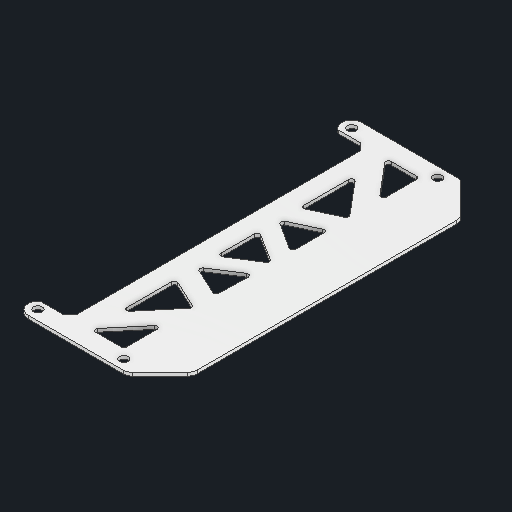
# Autodesk Inventor part: ramp
Saved by Autodesk Inventor 2025 (Build 290162000, 162)
## iProperties
Created: 2024-08-22
Part Number: ramp
Material: Acetal Resin, White
Document SubType Name: Sheet Metal
Designer: averey
Density: 1.425 g/cm^3
Appearance: Smooth - White
Flat Pattern Width: 6.82628 cm
Flat Pattern Length: 16.0338 cm
Flat Pattern Area: 109.451 cm^2
Sheet Metal Rule: Default
Sheet Metal Width: 2.688 in
Sheet Metal Length: 6.313 in
Sheet Metal Area: 16.965 in^2
Author: averey
Autodesk Inventor part; units mm, degrees
ref_plane "YZ Plane" through (0, 0, 0) normal (1, 0, 0) x (0, 1, 0)
ref_plane "XZ Plane" through (0, 0, 0) normal (0, 1, 0) x (-1, 0, 0)
ref_plane "XY Plane" through (0, 0, 0) normal (0, 0, 1) x (1, 0, 0)
sketch "Sketch1" plane through (0, 0, 0) normal (0, 1, 0) x (-1, 0, 0)
  circle A0 centre (0, 0) radius 2.0955
  circle A1 centre (41.2753, 0) radius 2.0955
  circle A2 centre (0, -150.8125) radius 2.0955
  circle A3 centre (41.2753, -150.8125) radius 2.0955
  arc A4 (43.9079, -3.9688) -> (41.2753, 4.7625) centre (41.2753, 0) ccw
  arc A5 (41.2753, -155.575) -> (43.9079, -146.8438) centre (41.2753, -150.8125) ccw
  line L0 (29.8453, -7.366) -> (29.8453, -143.4465)
  line L1 (41.2753, -155.575) -> (0, -155.575)
  line L2 (0, 4.7625) -> (41.2753, 4.7625)
  line L3 (33.2426, -3.9688) -> (29.8453, -7.366)
  line L4 (29.8453, -143.4465) -> (33.2426, -146.8438)
  line L5 (17.9778, -146.431) -> (5.6515, -146.431)
  line L6 (5.6515, -4.3815) -> (17.9778, -4.3815)
  line L7 (18.9507, -6.4678) -> (6.6244, -21.1577)
  line L8 (20.7013, -4.3815) -> (39.8776, -4.3815) construction
  line L9 (18.4584, -21.28) -> (5.4454, -36.7883)
  line L10 (5.8815, -38.7557) -> (18.8946, -44.8238)
  line L11 (4.3815, -38.0562) -> (18.7398, -38.0562) construction
  line L12 (18.6151, -54.7828) -> (6.3567, -49.0665)
  line L13 (6.1698, -65.111) -> (18.7659, -57.0016)
  line L14 (18.9507, -144.3447) -> (6.6244, -129.6548)
  line L15 (20.7013, -146.431) -> (39.8776, -146.431) construction
  line L16 (18.4584, -129.5325) -> (5.4454, -114.0242)
  line L17 (5.8815, -112.0568) -> (18.8946, -105.9887)
  line L18 (4.3815, -112.7563) -> (18.7398, -112.7563) construction
  line L19 (18.6151, -96.0297) -> (6.1882, -101.8245)
  line L20 (18.7659, -93.8109) -> (6.339, -85.8105)
  line L21 (20.7013, -95.0569) -> (35.4808, -95.0569) construction
  line L22 (6.0792, -76.4797) -> (18.7526, -84.4929)
  line L23 (6.0792, -74.3328) -> (18.7526, -66.3196)
  line L24 (4.3815, -20.3414) -> (4.3815, -5.6515)
  line L25 (20.7013, -22.0963) -> (20.7013, -43.6728)
  line L26 (4.2127, -64.0121) -> (4.5503, -50.1866)
  line L27 (20.7013, -67.3931) -> (20.7013, -83.4194)
  line L28 (20.7013, -107.1397) -> (20.7013, -128.7162)
  line L29 (4.3815, -145.161) -> (4.3815, -130.4711)
  line L30 (4.3815, -100.6735) -> (4.3815, -86.8783)
  arc A6 (4.3815, -20.3414) -> (6.6244, -21.1577) centre (5.6515, -20.3414) ccw
  arc A7 (5.6515, -4.3815) -> (4.3815, -5.6515) centre (5.6515, -5.6515) ccw
  arc A8 (18.9507, -6.4678) -> (17.9778, -4.3815) centre (17.9778, -5.6515) ccw
  arc A9 (20.7013, -22.0963) -> (18.4584, -21.28) centre (19.4313, -22.0963) ccw
  arc A10 (5.4454, -36.7883) -> (5.8815, -38.7557) centre (6.4183, -37.6047) ccw
  arc A11 (18.8946, -44.8238) -> (20.7013, -43.6728) centre (19.4313, -43.6728) ccw
  arc A12 (6.3567, -49.0665) -> (4.5503, -50.1866) centre (5.8199, -50.2176) ccw
  arc A13 (4.2127, -64.0121) -> (6.1698, -65.111) centre (5.4823, -64.0431) ccw
  arc A14 (18.7659, -57.0016) -> (18.6151, -54.7828) centre (18.0784, -55.9338) ccw
  arc A15 (6.0792, -74.3328) -> (6.0792, -76.4797) centre (6.7579, -75.4063) ccw
  arc A16 (18.7526, -84.4929) -> (20.7013, -83.4194) centre (19.4313, -83.4194) ccw
  arc A17 (20.7013, -67.3931) -> (18.7526, -66.3196) centre (19.4313, -67.3931) ccw
  arc A18 (6.339, -85.8105) -> (4.3815, -86.8783) centre (5.6515, -86.8783) ccw
  arc A19 (18.6151, -96.0297) -> (18.7659, -93.8109) centre (18.0784, -94.8787) ccw
  arc A20 (4.3815, -100.6735) -> (6.1882, -101.8245) centre (5.6515, -100.6735) ccw
  arc A21 (20.7013, -107.1397) -> (18.8946, -105.9887) centre (19.4313, -107.1397) ccw
  arc A22 (5.8815, -112.0568) -> (5.4454, -114.0242) centre (6.4183, -113.2078) ccw
  arc A23 (18.4584, -129.5325) -> (20.7013, -128.7162) centre (19.4313, -128.7162) ccw
  arc A24 (6.6244, -129.6548) -> (4.3815, -130.4711) centre (5.6515, -130.4711) ccw
  arc A25 (4.3815, -145.161) -> (5.6515, -146.431) centre (5.6515, -145.161) ccw
  arc A26 (17.9778, -146.431) -> (18.9507, -144.3447) centre (17.9778, -145.161) ccw
  line L31 (0, 4.7625) -> (-4.3773, 4.7625)
  line L32 (-22.225, -13.0852) -> (-22.225, -137.7273)
  line L33 (-4.3773, -155.575) -> (0, -155.575)
  line L34 (43.9079, -3.9688) -> (33.2426, -3.9688)
  line L35 (43.9079, -146.8438) -> (33.2426, -146.8438)
  line L36 (-20.8301, -9.7176) -> (-7.7449, 3.3676)
  line L37 (-20.8301, -141.0949) -> (-7.7449, -154.1801)
  arc A27 (-4.3773, 4.7625) -> (-7.7449, 3.3676) centre (-4.3773, 0) ccw
  arc A28 (-20.8301, -9.7176) -> (-22.225, -13.0852) centre (-17.4625, -13.0852) ccw
  arc A29 (-22.225, -137.7273) -> (-20.8301, -141.0949) centre (-17.4625, -137.7273) ccw
  arc A30 (-7.7449, -154.1801) -> (-4.3773, -155.575) centre (-4.3773, -150.8125) ccw
  point P0 (29.8453, -4.7625)
  point P1 (29.8453, -146.05)
  point P2 (32.8298, -4.3815)
  point P3 (32.4488, -146.05)
  point P4 (-17.4625, 4.7625)
  point P5 (-22.225, 0)
  point P6 (-17.4625, -155.575)
  point P7 (-22.225, -150.8125)
  point P8 (-22.225, 4.7625)
  point P9 (-22.225, -11.1125)
  point P10 (-6.35, 4.7625)
  point P11 (-22.225, 4.7625)
  point P12 (-22.225, -139.7)
  point P13 (-6.35, -155.575)
  point P14 (-22.225, -155.575)
  point P15 (4.3815, -57.0993)
  dimension "d0" = 4.191
  dimension "d3" = 9.525
  dimension "d20" = 1.27
  dimension "d24" = 22.225
  dimension "d27" = 15.875
  dimension "d28" = 15.875
  dimension "d29" = 15.875
  dimension "d30" = 15.875
  dimension "d31" = 4.7625
  constraints: 74 end point, 54 point on circle, 50 tangent, 31 centre point, 26 point on line, 23 equal radius, 12 horizontal, 6 vertical, 5 equal length, 3 coincident, 3 parallel, 1 midpoint, 28 other
  measures "d0" diameter of A0
  measures "d3" diameter of A4
  measures "d20" radius of A6
  measures "d27" distance of point (-22.225, -11.113) point (-22.225, 4.762)
  measures "d28" distance of point (-6.35, 4.762) point (-22.225, 4.762)
  measures "d29" distance of point (-22.225, -139.7) point (-22.225, -155.575)
  measures "d30" distance of point (-6.35, -155.575) point (-22.225, -155.575)
  measures "d31" radius of A27
extrude "Extrusion1" add sketch "Sketch1" along normal blind 1.5875
equation "\"d28\" = d27"
equation "\"d29\" = d27"
equation "\"d30\" = d29"
equation "\"BendRadius\" = Thickness"
equation "\"BendReliefWidth\" = Thickness"
equation "\"BendReliefDepth\" = 0.5 * Thickness"
equation "\"CornerReliefSize\" = 4 * Thickness"
equation "\"MinimumRemnant\" = 2 * Thickness"
equation "\"TransitionRadius\" = BendRadius"
equation "\"JacobiRadiusSize\" = BendRadius"
equation "\"GapSize\" = Thickness"
equation "\"Thickness\" = 1.5875"
body "Solid1"
